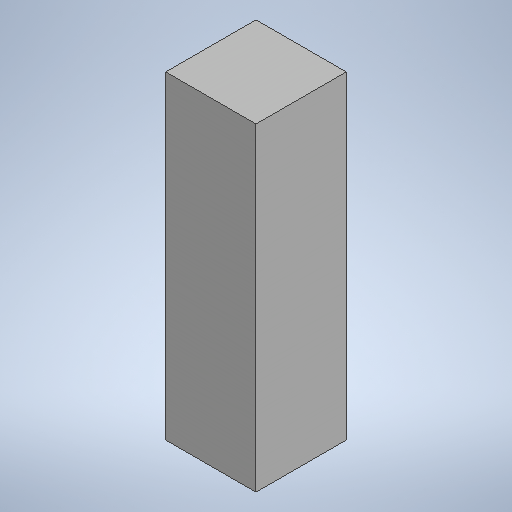
# Autodesk Inventor part: Pier
Saved by Autodesk Inventor 2025 (Build 290162010, 162A)
## iProperties
Created: 2024-08-07
Part Number: Pier
Material: Concrete
Document SubType Name: Modeling
Designer: Tom
Density: 2.40731 g/cm^3
Appearance: Light Gray
Author: Tom
Autodesk Inventor part; units mm, degrees
ref_plane "YZ Plane" through (0, 0, 0) normal (1, 0, 0) x (0, 1, 0)
ref_plane "XZ Plane" through (0, 0, 0) normal (0, 1, 0) x (-1, 0, 0)
ref_plane "XY Plane" through (0, 0, 0) normal (0, 0, 1) x (1, 0, 0)
sketch "Sketch1" plane through (0, 0, 0) normal (0, 1, 0) x (-1, 0, 0)
  line L0 (177.8, -177.8) -> (-177.8, -177.8)
  line L1 (-177.8, -177.8) -> (-177.8, 177.8)
  line L2 (-177.8, 177.8) -> (177.8, 177.8)
  line L3 (177.8, 177.8) -> (177.8, -177.8)
  line L4 (0, -177.8) -> (0, 177.8)
  line L5 (-177.8, 0) -> (177.8, 0)
  point P0 (0, 0)
  point P1 (0, 0)
  dimension "d3" = 355.6
  constraints: 12 end point, 5 midpoint, 2 parallel, 2 perpendicular, 1 coincident, 1 horizontal
  measures "d3" distance of L0.start L0.end
extrude "Extrusion1" add sketch "Sketch1" along normal blind 1256.5063
body "Solid1"
